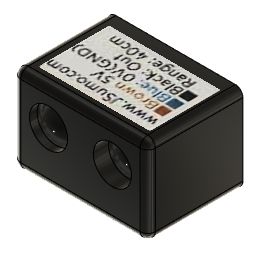
JS40F v1 (Autodesk Fusion 360 design; units mm, degrees)
Autodesk Fusion 360 part; units mm, degrees
sketch "Boceto1" plane through (0, 0, 0) normal (0, 1, 0) x (1, 0, 0)
  line L0 (-8.85, 0) -> (-8.85, -5.75)
  line L1 (-8.85, -5.75) -> (8.85, -5.75)
  line L2 (8.85, -5.75) -> (8.85, 5.75)
  line L3 (8.85, 5.75) -> (-8.85, 5.75)
  line L4 (-8.85, 5.75) -> (-8.85, 0)
  dimension "d1" = 8.85
  dimension "d2" = 5.75
  dimension "d3" = 17.7
  dimension "d4" = 11.5
  dimension "d5" = 17.7
  constraint perpendicular L0 L1
  constraint perpendicular L1 L2
  constraint perpendicular L2 L3
  measures "d1" distance of origin L0.start
  measures "d2" distance of L0.start L0.end
  measures "d3" distance of L0.end L1.end
  measures "d4" distance of L1.end L2.end
  measures "d5" distance of L2.end L3.end
extrude "Extruir1" add sketch "Boceto1" along normal blind 12.5
sketch "Boceto2" plane through (0, 0, 0) normal (0, -1, 0) x (1, 0, 0)
  line L0 (-8.85, 5.75) -> (-8.85, -5.75)
  line L1 (-8.85, -5.75) -> (8.85, -5.75)
  line L2 (8.85, -5.75) -> (8.85, 5.75)
  line L3 (8.85, 5.75) -> (-8.85, 5.75)
  line L4 (8.85, -5.75) -> (4.195, -5.75)
  line L5 (4.195, -5.75) -> (-4.195, -5.75)
  line L6 (4.195, -5.75) -> (4.195, 1.04)
  line L7 (-4.195, -5.75) -> (-4.195, 1.04)
  circle A0 centre (4.195, 1.04) radius 2.5
  circle A1 centre (-4.195, 1.04) radius 2.5
  dimension "d8" = 4.655
  dimension "d9" = 8.39
  dimension "d10" = 6.79
  dimension "d11" = 6.79
  dimension "d12" = 5
  dimension "d13" = 5
  constraint coincident L1.end L2.start
  constraint perpendicular L2 L4
  constraint parallel L1 L5
  constraint perpendicular L4 L6
  constraint perpendicular L5 L7
  constraint coincident L6.end A0.centre
  constraint coincident L7.end A1.centre
  measures "d8" distance of L1.end L4.end
  measures "d9" distance of L4.end L5.end
  measures "d10" distance of L4.end L6.end
  measures "d11" distance of L5.end L7.end
  measures "d12" diameter of A0
  measures "d13" diameter of A1
extrude "Extruir2" cut sketch "Boceto2" against normal blind 7 contours A0
extrude "Extruir3" cut sketch "Boceto2" against normal blind 7 contours A1
fillet "Empalme1" radius 1 3 edges at (8.85, 6.25, 5.75) (0, 0, 5.75) (8.85, 0, 0)
fillet "Empalme2" radius 1 3 edges at (-8.85, 0, -0.5) (-8.85, 0.2929, 5.4571) (-8.85, 6.75, 5.75)
fillet "Empalme3" radius 1 5 edges at (8.85, 6.75, -5.75) (8.5571, 0.2929, -5.75) (0, 0, -5.75) (-8.5571, 0.2929, -5.75) (-8.85, 6.75, -5.75)
extrude "Extruir4" add 1 faces at (4.9913, 7, -0.2658) along direction (0, -1, 0) blind 3
extrude "Extruir5" add 1 faces at (-4.4262, 7, 0.3911) along direction (0, -1, 0) blind 4
fillet "Empalme4" radius 2 1 faces at (4.9913, 4, -0.2658)
fillet "Empalme5" radius 2 1 faces at (-4.4262, 3, 0.3911)
named bodies: "Body"
